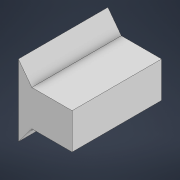
# Autodesk Inventor part: LinearSlider
Saved by Autodesk Inventor 2021 (Build 250183000, 183)
## iProperties
Created: 2021-01-30
Part Number: LinearSlider
Material: Generic
Document SubType Name: Modeling
Designer: argon
Density: 1 g/cm^3
Appearance: Default
Author: argon
Autodesk Inventor part; units mm, degrees
ref_plane "YZ Plane" through (0, 0, 0) normal (1, 0, 0) x (0, 1, 0)
ref_plane "XZ Plane" through (0, 0, 0) normal (0, 1, 0) x (-1, 0, 0)
ref_plane "XY Plane" through (0, 0, 0) normal (0, 0, 1) x (1, 0, 0)
sketch "Sketch1" plane through (0, 0, 0) normal (0, 0, 1) x (1, 0, 0)
  line L0 (-3, 3) -> (3, -3) construction
  line L1 (3, 3) -> (-3, -3) construction
  line L2 (0, 1) -> (3, 1)
  line L3 (3, 1) -> (3, -1)
  line L4 (3, -1) -> (0, -1)
  line L5 (0, -1) -> (0, 1)
  line L6 (0, 1) -> (3, -1) construction
  line L7 (3, 1) -> (0, -1) construction
  line L8 (0, 1) -> (0, 2)
  line L9 (0, 2) -> (1.5, 0)
  line L10 (0, -1) -> (0, -2)
  line L11 (0, -2) -> (1.5, 0)
  point P0 (0, 0)
  point P1 (0, 0)
  point P2 (0.75, 1)
  point P3 (0.75, -1)
  dimension "d0" = 6
  dimension "d1" = 2
  dimension "d2" = 3
  dimension "d3" = 1
  constraints: 24 end point, 4 midpoint, 2 parallel, 2 vertical, 1 equal length, 1 horizontal, 1 horizontal alignment, 1 perpendicular
  measures "d0" distance of L0.start L1.start
  measures "d1" distance of L4.end L2.start
  measures "d2" distance of L3.end L4.end
  measures "d3" distance of L4.end L10.end
extrude "Extrusion1" add sketch "Sketch1" along normal blind 5
body "Solid1"
